Autodesk Fusion 360 part; units mm, degrees
(part 11 of 14)
  line L7370 (-262.9775, 77.7875) -> (-273.976, 77.7875)
  line L7371 (-273.976, 77.7875) -> (-279.4753, 68.2625)
  line L7372 (-279.4753, 68.2625) -> (-273.976, 58.7375)
  line L7373 (-273.976, 58.7375) -> (-262.9775, 58.7375)
  line L7374 (-257.4782, 68.2625) -> (-262.9775, 77.7875)
  line L7375 (-262.9775, 58.7375) -> (-257.4782, 68.2625)
  line L7376 (-243.7301, 88.9) -> (-254.7286, 88.9)
  line L7377 (-254.7286, 88.9) -> (-260.2278, 79.375)
  line L7378 (-260.2278, 79.375) -> (-254.7286, 69.85)
  line L7379 (-254.7286, 69.85) -> (-243.7301, 69.85)
  line L7380 (-238.2308, 79.375) -> (-243.7301, 88.9)
  line L7381 (-243.7301, 69.85) -> (-238.2308, 79.375)
  line L7382 (-224.4826, 100.0125) -> (-235.4812, 100.0125)
  line L7383 (-235.4812, 100.0125) -> (-240.9804, 90.4875)
  line L7384 (-240.9804, 90.4875) -> (-235.4812, 80.9625)
  line L7385 (-235.4812, 80.9625) -> (-224.4826, 80.9625)
  line L7386 (-218.9834, 90.4875) -> (-224.4826, 100.0125)
  line L7387 (-224.4826, 80.9625) -> (-218.9834, 90.4875)
  line L7388 (-205.2352, 111.125) -> (-216.2337, 111.125)
  line L7389 (-216.2337, 111.125) -> (-221.733, 101.6)
  line L7390 (-221.733, 101.6) -> (-216.2337, 92.075)
  line L7391 (-216.2337, 92.075) -> (-205.2352, 92.075)
  line L7392 (-199.736, 101.6) -> (-205.2352, 111.125)
  line L7393 (-205.2352, 92.075) -> (-199.736, 101.6)
  line L7394 (-185.9878, 122.2375) -> (-196.9863, 122.2375)
  line L7395 (-196.9863, 122.2375) -> (-202.4856, 112.7125)
  line L7396 (-202.4856, 112.7125) -> (-196.9863, 103.1875)
  line L7397 (-196.9863, 103.1875) -> (-185.9878, 103.1875)
  line L7398 (-180.4886, 112.7125) -> (-185.9878, 122.2375)
  line L7399 (-185.9878, 103.1875) -> (-180.4886, 112.7125)
  line L7400 (-166.7404, 133.35) -> (-177.7389, 133.35)
  line L7401 (-177.7389, 133.35) -> (-183.2382, 123.825)
  line L7402 (-183.2382, 123.825) -> (-177.7389, 114.3)
  line L7403 (-177.7389, 114.3) -> (-166.7404, 114.3)
  line L7404 (-161.2411, 123.825) -> (-166.7404, 133.35)
  line L7405 (-166.7404, 114.3) -> (-161.2411, 123.825)
  line L7406 (-147.493, 144.4625) -> (-158.4915, 144.4625)
  line L7407 (-158.4915, 144.4625) -> (-163.9908, 134.9375)
  line L7408 (-163.9908, 134.9375) -> (-158.4915, 125.4125)
  line L7409 (-158.4915, 125.4125) -> (-147.493, 125.4125)
  line L7410 (-141.9937, 134.9375) -> (-147.493, 144.4625)
  line L7411 (-147.493, 125.4125) -> (-141.9937, 134.9375)
  line L7412 (-128.2456, 155.575) -> (-139.2441, 155.575)
  line L7413 (-139.2441, 155.575) -> (-144.7434, 146.05)
  line L7414 (-144.7434, 146.05) -> (-139.2441, 136.525)
  line L7415 (-139.2441, 136.525) -> (-128.2456, 136.525)
  line L7416 (-122.7463, 146.05) -> (-128.2456, 155.575)
  line L7417 (-128.2456, 136.525) -> (-122.7463, 146.05)
  line L7418 (-108.9982, 166.6875) -> (-119.9967, 166.6875)
  line L7419 (-119.9967, 166.6875) -> (-125.4959, 157.1625)
  line L7420 (-125.4959, 157.1625) -> (-119.9967, 147.6375)
  line L7421 (-119.9967, 147.6375) -> (-108.9982, 147.6375)
  line L7422 (-103.4989, 157.1625) -> (-108.9982, 166.6875)
  line L7423 (-108.9982, 147.6375) -> (-103.4989, 157.1625)
  line L7424 (-89.7507, 177.8) -> (-100.7493, 177.8)
  line L7425 (-100.7493, 177.8) -> (-106.2485, 168.275)
  line L7426 (-106.2485, 168.275) -> (-100.7493, 158.75)
  line L7427 (-100.7493, 158.75) -> (-89.7507, 158.75)
  line L7428 (-84.2515, 168.275) -> (-89.7507, 177.8)
  line L7429 (-89.7507, 158.75) -> (-84.2515, 168.275)
  line L7430 (-70.5033, 188.9125) -> (-81.5018, 188.9125)
  line L7431 (-81.5018, 188.9125) -> (-87.0011, 179.3875)
  line L7432 (-87.0011, 179.3875) -> (-81.5018, 169.8625)
  line L7433 (-81.5018, 169.8625) -> (-70.5033, 169.8625)
  line L7434 (-65.0041, 179.3875) -> (-70.5033, 188.9125)
  line L7435 (-70.5033, 169.8625) -> (-65.0041, 179.3875)
  line L7436 (-51.2559, 200.025) -> (-62.2544, 200.025)
  line L7437 (-62.2544, 200.025) -> (-67.7537, 190.5)
  line L7438 (-67.7537, 190.5) -> (-62.2544, 180.975)
  line L7439 (-62.2544, 180.975) -> (-51.2559, 180.975)
  line L7440 (-45.7566, 190.5) -> (-51.2559, 200.025)
  line L7441 (-51.2559, 180.975) -> (-45.7566, 190.5)
  line L7442 (-32.0085, 211.1375) -> (-43.007, 211.1375)
  line L7443 (-43.007, 211.1375) -> (-48.5063, 201.6125)
  line L7444 (-48.5063, 201.6125) -> (-43.007, 192.0875)
  line L7445 (-43.007, 192.0875) -> (-32.0085, 192.0875)
  line L7446 (-26.5092, 201.6125) -> (-32.0085, 211.1375)
  line L7447 (-32.0085, 192.0875) -> (-26.5092, 201.6125)
  line L7448 (-12.7611, 222.25) -> (-23.7596, 222.25)
  line L7449 (-23.7596, 222.25) -> (-29.2589, 212.725)
  line L7450 (-29.2589, 212.725) -> (-23.7596, 203.2)
  line L7451 (-23.7596, 203.2) -> (-12.7611, 203.2)
  line L7452 (-7.2618, 212.725) -> (-12.7611, 222.25)
  line L7453 (-12.7611, 203.2) -> (-7.2618, 212.725)
  line L7454 (6.4863, 233.3625) -> (-4.5122, 233.3625)
  line L7455 (-4.5122, 233.3625) -> (-10.0114, 223.8375)
  line L7456 (-10.0114, 223.8375) -> (-4.5122, 214.3125)
  line L7457 (-4.5122, 214.3125) -> (6.4863, 214.3125)
  line L7458 (11.9856, 223.8375) -> (6.4863, 233.3625)
  line L7459 (6.4863, 214.3125) -> (11.9856, 223.8375)
  line L7460 (25.7337, 244.475) -> (14.7352, 244.475)
  line L7461 (14.7352, 244.475) -> (9.236, 234.95)
  line L7462 (9.236, 234.95) -> (14.7352, 225.425)
  line L7463 (14.7352, 225.425) -> (25.7337, 225.425)
  line L7464 (31.233, 234.95) -> (25.7337, 244.475)
  line L7465 (25.7337, 225.425) -> (31.233, 234.95)
  line L7466 (44.9812, 255.5875) -> (33.9826, 255.5875)
  line L7467 (33.9826, 255.5875) -> (28.4834, 246.0625)
  line L7468 (28.4834, 246.0625) -> (33.9826, 236.5375)
  line L7469 (33.9826, 236.5375) -> (44.9812, 236.5375)
  line L7470 (50.4804, 246.0625) -> (44.9812, 255.5875)
  line L7471 (44.9812, 236.5375) -> (50.4804, 246.0625)
  line L7472 (64.2286, 266.7) -> (53.2301, 266.7)
  line L7473 (53.2301, 266.7) -> (47.7308, 257.175)
  line L7474 (47.7308, 257.175) -> (53.2301, 247.65)
  line L7475 (53.2301, 247.65) -> (64.2286, 247.65)
  line L7476 (69.7278, 257.175) -> (64.2286, 266.7)
  line L7477 (64.2286, 247.65) -> (69.7278, 257.175)
  line L7478 (83.476, 277.8125) -> (72.4775, 277.8125)
  line L7479 (72.4775, 277.8125) -> (66.9782, 268.2875)
  line L7480 (66.9782, 268.2875) -> (72.4775, 258.7625)
  line L7481 (72.4775, 258.7625) -> (83.476, 258.7625)
  line L7482 (88.9753, 268.2875) -> (83.476, 277.8125)
  line L7483 (83.476, 258.7625) -> (88.9753, 268.2875)
  line L7484 (102.7234, 288.925) -> (91.7249, 288.925)
  line L7485 (91.7249, 288.925) -> (86.2256, 279.4)
  line L7486 (86.2256, 279.4) -> (91.7249, 269.875)
  line L7487 (91.7249, 269.875) -> (102.7234, 269.875)
  line L7488 (108.2227, 279.4) -> (102.7234, 288.925)
  line L7489 (102.7234, 269.875) -> (108.2227, 279.4)
  line L7490 (121.9708, 300.0375) -> (110.9723, 300.0375)
  line L7491 (110.9723, 300.0375) -> (105.473, 290.5125)
  line L7492 (105.473, 290.5125) -> (110.9723, 280.9875)
  line L7493 (110.9723, 280.9875) -> (121.9708, 280.9875)
  line L7494 (127.4701, 290.5125) -> (121.9708, 300.0375)
  line L7495 (121.9708, 280.9875) -> (127.4701, 290.5125)
  line L7496 (141.2182, 311.15) -> (130.2197, 311.15)
  line L7497 (130.2197, 311.15) -> (124.7205, 301.625)
  line L7498 (124.7205, 301.625) -> (130.2197, 292.1)
  line L7499 (130.2197, 292.1) -> (141.2182, 292.1)
  line L7500 (146.7175, 301.625) -> (141.2182, 311.15)
  line L7501 (141.2182, 292.1) -> (146.7175, 301.625)
  line L7502 (160.4657, 322.2625) -> (149.4671, 322.2625)
  line L7503 (149.4671, 322.2625) -> (143.9679, 312.7375)
  line L7504 (143.9679, 312.7375) -> (149.4671, 303.2125)
  line L7505 (149.4671, 303.2125) -> (160.4657, 303.2125)
  line L7506 (165.9649, 312.7375) -> (160.4657, 322.2625)
  line L7507 (160.4657, 303.2125) -> (165.9649, 312.7375)
  line L7508 (179.7131, 333.375) -> (168.7145, 333.375)
  line L7509 (168.7145, 333.375) -> (163.2153, 323.85)
  line L7510 (163.2153, 323.85) -> (168.7145, 314.325)
  line L7511 (168.7145, 314.325) -> (179.7131, 314.325)
  line L7512 (185.2123, 323.85) -> (179.7131, 333.375)
  line L7513 (179.7131, 314.325) -> (185.2123, 323.85)
  line L7514 (198.9605, 344.4875) -> (187.962, 344.4875)
  line L7515 (187.962, 344.4875) -> (182.4627, 334.9625)
  line L7516 (182.4627, 334.9625) -> (187.962, 325.4375)
  line L7517 (187.962, 325.4375) -> (198.9605, 325.4375)
  line L7518 (204.4597, 334.9625) -> (198.9605, 344.4875)
  line L7519 (198.9605, 325.4375) -> (204.4597, 334.9625)
  line L7520 (218.2079, 355.6) -> (207.2094, 355.6)
  line L7521 (207.2094, 355.6) -> (201.7101, 346.075)
  line L7522 (201.7101, 346.075) -> (207.2094, 336.55)
  line L7523 (207.2094, 336.55) -> (218.2079, 336.55)
  line L7524 (223.7072, 346.075) -> (218.2079, 355.6)
  line L7525 (218.2079, 336.55) -> (223.7072, 346.075)
  line L7526 (237.4553, 366.7125) -> (226.4568, 366.7125)
  line L7527 (226.4568, 366.7125) -> (220.9575, 357.1875)
  line L7528 (220.9575, 357.1875) -> (226.4568, 347.6625)
  line L7529 (226.4568, 347.6625) -> (237.4553, 347.6625)
  line L7530 (242.9546, 357.1875) -> (237.4553, 366.7125)
  line L7531 (237.4553, 347.6625) -> (242.9546, 357.1875)
  line L7532 (256.7027, 377.825) -> (245.7042, 377.825)
  line L7533 (245.7042, 377.825) -> (240.2049, 368.3)
  line L7534 (240.2049, 368.3) -> (245.7042, 358.775)
  line L7535 (245.7042, 358.775) -> (256.7027, 358.775)
  line L7536 (262.202, 368.3) -> (256.7027, 377.825)
  line L7537 (256.7027, 358.775) -> (262.202, 368.3)
  line L7538 (275.9501, 388.9375) -> (264.9516, 388.9375)
  line L7539 (264.9516, 388.9375) -> (259.4524, 379.4125)
  line L7540 (259.4524, 379.4125) -> (264.9516, 369.8875)
  line L7541 (264.9516, 369.8875) -> (275.9501, 369.8875)
  line L7542 (281.4494, 379.4125) -> (275.9501, 388.9375)
  line L7543 (275.9501, 369.8875) -> (281.4494, 379.4125)
  line L7544 (295.1976, 400.05) -> (284.199, 400.05)
  line L7545 (284.199, 400.05) -> (278.6998, 390.525)
  line L7546 (278.6998, 390.525) -> (284.199, 381)
  line L7547 (284.199, 381) -> (295.1976, 381)
  line L7548 (300.6968, 390.525) -> (295.1976, 400.05)
  line L7549 (295.1976, 381) -> (300.6968, 390.525)
  line L7550 (314.445, 411.1625) -> (303.4464, 411.1625)
  line L7551 (303.4464, 411.1625) -> (297.9472, 401.6375)
  line L7552 (297.9472, 401.6375) -> (303.4464, 392.1125)
  line L7553 (303.4464, 392.1125) -> (314.445, 392.1125)
  line L7554 (319.9442, 401.6375) -> (314.445, 411.1625)
  line L7555 (314.445, 392.1125) -> (319.9442, 401.6375)
  line L7556 (333.6924, 422.275) -> (322.6939, 422.275)
  line L7557 (322.6939, 422.275) -> (317.1946, 412.75)
  line L7558 (317.1946, 412.75) -> (322.6939, 403.225)
  line L7559 (322.6939, 403.225) -> (333.6924, 403.225)
  line L7560 (339.1916, 412.75) -> (333.6924, 422.275)
  line L7561 (333.6924, 403.225) -> (339.1916, 412.75)
  line L7562 (352.9398, 433.3875) -> (341.9413, 433.3875)
  line L7563 (341.9413, 433.3875) -> (336.442, 423.8625)
  line L7564 (336.442, 423.8625) -> (341.9413, 414.3375)
  line L7565 (341.9413, 414.3375) -> (352.9398, 414.3375)
  line L7566 (358.4391, 423.8625) -> (352.9398, 433.3875)
  line L7567 (352.9398, 414.3375) -> (358.4391, 423.8625)
  line L7568 (372.1872, 444.5) -> (361.1887, 444.5)
  line L7569 (361.1887, 444.5) -> (355.6894, 434.975)
  line L7570 (355.6894, 434.975) -> (361.1887, 425.45)
  line L7571 (361.1887, 425.45) -> (372.1872, 425.45)
  line L7572 (377.6865, 434.975) -> (372.1872, 444.5)
  line L7573 (372.1872, 425.45) -> (377.6865, 434.975)
  line L7574 (-782.6577, -200.025) -> (-793.6562, -200.025)
  line L7575 (-793.6562, -200.025) -> (-799.1554, -209.55)
  line L7576 (-799.1554, -209.55) -> (-793.6562, -219.075)
  line L7577 (-793.6562, -219.075) -> (-782.6577, -219.075)
  line L7578 (-777.1584, -209.55) -> (-782.6577, -200.025)
  line L7579 (-782.6577, -219.075) -> (-777.1584, -209.55)
  line L7580 (-763.4102, -188.9125) -> (-774.4088, -188.9125)
  line L7581 (-774.4088, -188.9125) -> (-779.908, -198.4375)
  line L7582 (-779.908, -198.4375) -> (-774.4088, -207.9625)
  line L7583 (-774.4088, -207.9625) -> (-763.4102, -207.9625)
  line L7584 (-757.911, -198.4375) -> (-763.4102, -188.9125)
  line L7585 (-763.4102, -207.9625) -> (-757.911, -198.4375)
  line L7586 (-744.1628, -177.8) -> (-755.1614, -177.8)
  line L7587 (-755.1614, -177.8) -> (-760.6606, -187.325)
  line L7588 (-760.6606, -187.325) -> (-755.1614, -196.85)
  line L7589 (-755.1614, -196.85) -> (-744.1628, -196.85)
  line L7590 (-738.6636, -187.325) -> (-744.1628, -177.8)
  line L7591 (-744.1628, -196.85) -> (-738.6636, -187.325)
  line L7592 (-724.9154, -166.6875) -> (-735.9139, -166.6875)
  line L7593 (-735.9139, -166.6875) -> (-741.4132, -176.2125)
  line L7594 (-741.4132, -176.2125) -> (-735.9139, -185.7375)
  line L7595 (-735.9139, -185.7375) -> (-724.9154, -185.7375)
  line L7596 (-719.4162, -176.2125) -> (-724.9154, -166.6875)
  line L7597 (-724.9154, -185.7375) -> (-719.4162, -176.2125)
  line L7598 (-705.668, -155.575) -> (-716.6665, -155.575)
  line L7599 (-716.6665, -155.575) -> (-722.1658, -165.1)
  line L7600 (-722.1658, -165.1) -> (-716.6665, -174.625)
  line L7601 (-716.6665, -174.625) -> (-705.668, -174.625)
  line L7602 (-700.1687, -165.1) -> (-705.668, -155.575)
  line L7603 (-705.668, -174.625) -> (-700.1687, -165.1)
  line L7604 (-686.4206, -144.4625) -> (-697.4191, -144.4625)
  line L7605 (-697.4191, -144.4625) -> (-702.9184, -153.9875)
  line L7606 (-702.9184, -153.9875) -> (-697.4191, -163.5125)
  line L7607 (-697.4191, -163.5125) -> (-686.4206, -163.5125)
  line L7608 (-680.9213, -153.9875) -> (-686.4206, -144.4625)
  line L7609 (-686.4206, -163.5125) -> (-680.9213, -153.9875)
  line L7610 (-667.1732, -133.35) -> (-678.1717, -133.35)
  line L7611 (-678.1717, -133.35) -> (-683.671, -142.875)
  line L7612 (-683.671, -142.875) -> (-678.1717, -152.4)
  line L7613 (-678.1717, -152.4) -> (-667.1732, -152.4)
  line L7614 (-661.6739, -142.875) -> (-667.1732, -133.35)
  line L7615 (-667.1732, -152.4) -> (-661.6739, -142.875)
  line L7616 (-647.9258, -122.2375) -> (-658.9243, -122.2375)
  line L7617 (-658.9243, -122.2375) -> (-664.4235, -131.7625)
  line L7618 (-664.4235, -131.7625) -> (-658.9243, -141.2875)
  line L7619 (-658.9243, -141.2875) -> (-647.9258, -141.2875)
  line L7620 (-642.4265, -131.7625) -> (-647.9258, -122.2375)
  line L7621 (-647.9258, -141.2875) -> (-642.4265, -131.7625)
  line L7622 (-628.6783, -111.125) -> (-639.6769, -111.125)
  line L7623 (-639.6769, -111.125) -> (-645.1761, -120.65)
  line L7624 (-645.1761, -120.65) -> (-639.6769, -130.175)
  line L7625 (-639.6769, -130.175) -> (-628.6783, -130.175)
  line L7626 (-623.1791, -120.65) -> (-628.6783, -111.125)
  line L7627 (-628.6783, -130.175) -> (-623.1791, -120.65)
  line L7628 (-609.4309, -100.0125) -> (-620.4295, -100.0125)
  line L7629 (-620.4295, -100.0125) -> (-625.9287, -109.5375)
  line L7630 (-625.9287, -109.5375) -> (-620.4295, -119.0625)
  line L7631 (-620.4295, -119.0625) -> (-609.4309, -119.0625)
  line L7632 (-603.9317, -109.5375) -> (-609.4309, -100.0125)
  line L7633 (-609.4309, -119.0625) -> (-603.9317, -109.5375)
  line L7634 (-590.1835, -88.9) -> (-601.182, -88.9)
  line L7635 (-601.182, -88.9) -> (-606.6813, -98.425)
  line L7636 (-606.6813, -98.425) -> (-601.182, -107.95)
  line L7637 (-601.182, -107.95) -> (-590.1835, -107.95)
  line L7638 (-584.6843, -98.425) -> (-590.1835, -88.9)
  line L7639 (-590.1835, -107.95) -> (-584.6843, -98.425)
  line L7640 (-570.9361, -77.7875) -> (-581.9346, -77.7875)
  line L7641 (-581.9346, -77.7875) -> (-587.4339, -87.3125)
  line L7642 (-587.4339, -87.3125) -> (-581.9346, -96.8375)
  line L7643 (-581.9346, -96.8375) -> (-570.9361, -96.8375)
  line L7644 (-565.4368, -87.3125) -> (-570.9361, -77.7875)
  line L7645 (-570.9361, -96.8375) -> (-565.4368, -87.3125)
  line L7646 (-551.6887, -66.675) -> (-562.6872, -66.675)
  line L7647 (-562.6872, -66.675) -> (-568.1865, -76.2)
  line L7648 (-568.1865, -76.2) -> (-562.6872, -85.725)
  line L7649 (-562.6872, -85.725) -> (-551.6887, -85.725)
  line L7650 (-546.1894, -76.2) -> (-551.6887, -66.675)
  line L7651 (-551.6887, -85.725) -> (-546.1894, -76.2)
  line L7652 (-532.4413, -55.5625) -> (-543.4398, -55.5625)
  line L7653 (-543.4398, -55.5625) -> (-548.9391, -65.0875)
  line L7654 (-548.9391, -65.0875) -> (-543.4398, -74.6125)
  line L7655 (-543.4398, -74.6125) -> (-532.4413, -74.6125)
  line L7656 (-526.942, -65.0875) -> (-532.4413, -55.5625)
  line L7657 (-532.4413, -74.6125) -> (-526.942, -65.0875)
  line L7658 (-513.1939, -44.45) -> (-524.1924, -44.45)
  line L7659 (-524.1924, -44.45) -> (-529.6916, -53.975)
  line L7660 (-529.6916, -53.975) -> (-524.1924, -63.5)
  line L7661 (-524.1924, -63.5) -> (-513.1939, -63.5)
  line L7662 (-507.6946, -53.975) -> (-513.1939, -44.45)
  line L7663 (-513.1939, -63.5) -> (-507.6946, -53.975)
  line L7664 (-493.9464, -33.3375) -> (-504.945, -33.3375)
  line L7665 (-504.945, -33.3375) -> (-510.4442, -42.8625)
  line L7666 (-510.4442, -42.8625) -> (-504.945, -52.3875)
  line L7667 (-504.945, -52.3875) -> (-493.9464, -52.3875)
  line L7668 (-488.4472, -42.8625) -> (-493.9464, -33.3375)
  line L7669 (-493.9464, -52.3875) -> (-488.4472, -42.8625)
  line L7670 (-474.699, -22.225) -> (-485.6976, -22.225)
  line L7671 (-485.6976, -22.225) -> (-491.1968, -31.75)
  line L7672 (-491.1968, -31.75) -> (-485.6976, -41.275)
  line L7673 (-485.6976, -41.275) -> (-474.699, -41.275)
  line L7674 (-469.1998, -31.75) -> (-474.699, -22.225)
  line L7675 (-474.699, -41.275) -> (-469.1998, -31.75)
  line L7676 (-455.4516, -11.1125) -> (-466.4501, -11.1125)
  line L7677 (-466.4501, -11.1125) -> (-471.9494, -20.6375)
  line L7678 (-471.9494, -20.6375) -> (-466.4501, -30.1625)
  line L7679 (-466.4501, -30.1625) -> (-455.4516, -30.1625)
  line L7680 (-449.9524, -20.6375) -> (-455.4516, -11.1125)
  line L7681 (-455.4516, -30.1625) -> (-449.9524, -20.6375)
  line L7682 (-436.2042, 0) -> (-447.2027, 0)
  line L7683 (-447.2027, 0) -> (-452.702, -9.525)
  line L7684 (-452.702, -9.525) -> (-447.2027, -19.05)
  line L7685 (-447.2027, -19.05) -> (-436.2042, -19.05)
  line L7686 (-430.7049, -9.525) -> (-436.2042, 0)
  line L7687 (-436.2042, -19.05) -> (-430.7049, -9.525)
  line L7688 (-416.9568, 11.1125) -> (-427.9553, 11.1125)
  line L7689 (-427.9553, 11.1125) -> (-433.4546, 1.5875)
  line L7690 (-433.4546, 1.5875) -> (-427.9553, -7.9375)
  line L7691 (-427.9553, -7.9375) -> (-416.9568, -7.9375)
  line L7692 (-411.4575, 1.5875) -> (-416.9568, 11.1125)
  line L7693 (-416.9568, -7.9375) -> (-411.4575, 1.5875)
  line L7694 (-397.7094, 22.225) -> (-408.7079, 22.225)
  line L7695 (-408.7079, 22.225) -> (-414.2072, 12.7)
  line L7696 (-414.2072, 12.7) -> (-408.7079, 3.175)
  line L7697 (-408.7079, 3.175) -> (-397.7094, 3.175)
  line L7698 (-392.2101, 12.7) -> (-397.7094, 22.225)
  line L7699 (-397.7094, 3.175) -> (-392.2101, 12.7)
  line L7700 (-378.462, 33.3375) -> (-389.4605, 33.3375)
  line L7701 (-389.4605, 33.3375) -> (-394.9597, 23.8125)
  line L7702 (-394.9597, 23.8125) -> (-389.4605, 14.2875)
  line L7703 (-389.4605, 14.2875) -> (-378.462, 14.2875)
  line L7704 (-372.9627, 23.8125) -> (-378.462, 33.3375)
  line L7705 (-378.462, 14.2875) -> (-372.9627, 23.8125)
  line L7706 (-359.2145, 44.45) -> (-370.2131, 44.45)
  line L7707 (-370.2131, 44.45) -> (-375.7123, 34.925)
  line L7708 (-375.7123, 34.925) -> (-370.2131, 25.4)
  line L7709 (-370.2131, 25.4) -> (-359.2145, 25.4)
  line L7710 (-353.7153, 34.925) -> (-359.2145, 44.45)
  line L7711 (-359.2145, 25.4) -> (-353.7153, 34.925)
  line L7712 (-339.9671, 55.5625) -> (-350.9657, 55.5625)
  line L7713 (-350.9657, 55.5625) -> (-356.4649, 46.0375)
  line L7714 (-356.4649, 46.0375) -> (-350.9657, 36.5125)
  line L7715 (-350.9657, 36.5125) -> (-339.9671, 36.5125)
  line L7716 (-334.4679, 46.0375) -> (-339.9671, 55.5625)
  line L7717 (-339.9671, 36.5125) -> (-334.4679, 46.0375)
  line L7718 (-320.7197, 66.675) -> (-331.7182, 66.675)
  line L7719 (-331.7182, 66.675) -> (-337.2175, 57.15)
  line L7720 (-337.2175, 57.15) -> (-331.7182, 47.625)
  line L7721 (-331.7182, 47.625) -> (-320.7197, 47.625)
  line L7722 (-315.2205, 57.15) -> (-320.7197, 66.675)
  line L7723 (-320.7197, 47.625) -> (-315.2205, 57.15)
  line L7724 (-301.4723, 77.7875) -> (-312.4708, 77.7875)
  line L7725 (-312.4708, 77.7875) -> (-317.9701, 68.2625)
  line L7726 (-317.9701, 68.2625) -> (-312.4708, 58.7375)
  line L7727 (-312.4708, 58.7375) -> (-301.4723, 58.7375)
  line L7728 (-295.973, 68.2625) -> (-301.4723, 77.7875)
  line L7729 (-301.4723, 58.7375) -> (-295.973, 68.2625)
  line L7730 (-282.2249, 88.9) -> (-293.2234, 88.9)
  line L7731 (-293.2234, 88.9) -> (-298.7227, 79.375)
  line L7732 (-298.7227, 79.375) -> (-293.2234, 69.85)
  line L7733 (-293.2234, 69.85) -> (-282.2249, 69.85)
  line L7734 (-276.7256, 79.375) -> (-282.2249, 88.9)
  line L7735 (-282.2249, 69.85) -> (-276.7256, 79.375)
  line L7736 (-262.9775, 100.0125) -> (-273.976, 100.0125)
  line L7737 (-273.976, 100.0125) -> (-279.4753, 90.4875)
  line L7738 (-279.4753, 90.4875) -> (-273.976, 80.9625)
  line L7739 (-273.976, 80.9625) -> (-262.9775, 80.9625)
  line L7740 (-257.4782, 90.4875) -> (-262.9775, 100.0125)
  line L7741 (-262.9775, 80.9625) -> (-257.4782, 90.4875)
  line L7742 (-243.7301, 111.125) -> (-254.7286, 111.125)
  line L7743 (-254.7286, 111.125) -> (-260.2278, 101.6)
  line L7744 (-260.2278, 101.6) -> (-254.7286, 92.075)
  line L7745 (-254.7286, 92.075) -> (-243.7301, 92.075)
  line L7746 (-238.2308, 101.6) -> (-243.7301, 111.125)
  line L7747 (-243.7301, 92.075) -> (-238.2308, 101.6)
  line L7748 (-224.4826, 122.2375) -> (-235.4812, 122.2375)
  line L7749 (-235.4812, 122.2375) -> (-240.9804, 112.7125)
  line L7750 (-240.9804, 112.7125) -> (-235.4812, 103.1875)
  line L7751 (-235.4812, 103.1875) -> (-224.4826, 103.1875)
  line L7752 (-218.9834, 112.7125) -> (-224.4826, 122.2375)
  line L7753 (-224.4826, 103.1875) -> (-218.9834, 112.7125)
  line L7754 (-205.2352, 133.35) -> (-216.2337, 133.35)
  line L7755 (-216.2337, 133.35) -> (-221.733, 123.825)
  line L7756 (-221.733, 123.825) -> (-216.2337, 114.3)
  line L7757 (-216.2337, 114.3) -> (-205.2352, 114.3)
  line L7758 (-199.736, 123.825) -> (-205.2352, 133.35)
  line L7759 (-205.2352, 114.3) -> (-199.736, 123.825)
  line L7760 (-185.9878, 144.4625) -> (-196.9863, 144.4625)
  line L7761 (-196.9863, 144.4625) -> (-202.4856, 134.9375)
  line L7762 (-202.4856, 134.9375) -> (-196.9863, 125.4125)
  line L7763 (-196.9863, 125.4125) -> (-185.9878, 125.4125)
  line L7764 (-180.4886, 134.9375) -> (-185.9878, 144.4625)
  line L7765 (-185.9878, 125.4125) -> (-180.4886, 134.9375)
  line L7766 (-166.7404, 155.575) -> (-177.7389, 155.575)
  line L7767 (-177.7389, 155.575) -> (-183.2382, 146.05)
  line L7768 (-183.2382, 146.05) -> (-177.7389, 136.525)
  line L7769 (-177.7389, 136.525) -> (-166.7404, 136.525)
  line L7770 (-161.2411, 146.05) -> (-166.7404, 155.575)
  line L7771 (-166.7404, 136.525) -> (-161.2411, 146.05)
  line L7772 (-147.493, 166.6875) -> (-158.4915, 166.6875)
  line L7773 (-158.4915, 166.6875) -> (-163.9908, 157.1625)
  line L7774 (-163.9908, 157.1625) -> (-158.4915, 147.6375)
  line L7775 (-158.4915, 147.6375) -> (-147.493, 147.6375)
  line L7776 (-141.9937, 157.1625) -> (-147.493, 166.6875)
  line L7777 (-147.493, 147.6375) -> (-141.9937, 157.1625)
  line L7778 (-128.2456, 177.8) -> (-139.2441, 177.8)
  line L7779 (-139.2441, 177.8) -> (-144.7434, 168.275)
  line L7780 (-144.7434, 168.275) -> (-139.2441, 158.75)
  line L7781 (-139.2441, 158.75) -> (-128.2456, 158.75)
  line L7782 (-122.7463, 168.275) -> (-128.2456, 177.8)
  line L7783 (-128.2456, 158.75) -> (-122.7463, 168.275)
  line L7784 (-108.9982, 188.9125) -> (-119.9967, 188.9125)
  line L7785 (-119.9967, 188.9125) -> (-125.4959, 179.3875)
  line L7786 (-125.4959, 179.3875) -> (-119.9967, 169.8625)
  line L7787 (-119.9967, 169.8625) -> (-108.9982, 169.8625)
  line L7788 (-103.4989, 179.3875) -> (-108.9982, 188.9125)
  line L7789 (-108.9982, 169.8625) -> (-103.4989, 179.3875)
  line L7790 (-89.7507, 200.025) -> (-100.7493, 200.025)
  line L7791 (-100.7493, 200.025) -> (-106.2485, 190.5)
  line L7792 (-106.2485, 190.5) -> (-100.7493, 180.975)
  line L7793 (-100.7493, 180.975) -> (-89.7507, 180.975)
  line L7794 (-84.2515, 190.5) -> (-89.7507, 200.025)
  line L7795 (-89.7507, 180.975) -> (-84.2515, 190.5)
  line L7796 (-70.5033, 211.1375) -> (-81.5018, 211.1375)
  line L7797 (-81.5018, 211.1375) -> (-87.0011, 201.6125)
  line L7798 (-87.0011, 201.6125) -> (-81.5018, 192.0875)
  line L7799 (-81.5018, 192.0875) -> (-70.5033, 192.0875)
  line L7800 (-65.0041, 201.6125) -> (-70.5033, 211.1375)
  line L7801 (-70.5033, 192.0875) -> (-65.0041, 201.6125)
  line L7802 (-51.2559, 222.25) -> (-62.2544, 222.25)
  line L7803 (-62.2544, 222.25) -> (-67.7537, 212.725)
  line L7804 (-67.7537, 212.725) -> (-62.2544, 203.2)
  line L7805 (-62.2544, 203.2) -> (-51.2559, 203.2)
  line L7806 (-45.7566, 212.725) -> (-51.2559, 222.25)
  line L7807 (-51.2559, 203.2) -> (-45.7566, 212.725)
  line L7808 (-32.0085, 233.3625) -> (-43.007, 233.3625)
  line L7809 (-43.007, 233.3625) -> (-48.5063, 223.8375)
  line L7810 (-48.5063, 223.8375) -> (-43.007, 214.3125)
  line L7811 (-43.007, 214.3125) -> (-32.0085, 214.3125)
  line L7812 (-26.5092, 223.8375) -> (-32.0085, 233.3625)
  line L7813 (-32.0085, 214.3125) -> (-26.5092, 223.8375)
  line L7814 (-12.7611, 244.475) -> (-23.7596, 244.475)
  line L7815 (-23.7596, 244.475) -> (-29.2589, 234.95)
  line L7816 (-29.2589, 234.95) -> (-23.7596, 225.425)
  line L7817 (-23.7596, 225.425) -> (-12.7611, 225.425)
  line L7818 (-7.2618, 234.95) -> (-12.7611, 244.475)
  line L7819 (-12.7611, 225.425) -> (-7.2618, 234.95)
  line L7820 (6.4863, 255.5875) -> (-4.5122, 255.5875)
  line L7821 (-4.5122, 255.5875) -> (-10.0114, 246.0625)
  line L7822 (-10.0114, 246.0625) -> (-4.5122, 236.5375)
  line L7823 (-4.5122, 236.5375) -> (6.4863, 236.5375)
  line L7824 (11.9856, 246.0625) -> (6.4863, 255.5875)
  line L7825 (6.4863, 236.5375) -> (11.9856, 246.0625)
  line L7826 (25.7337, 266.7) -> (14.7352, 266.7)
  line L7827 (14.7352, 266.7) -> (9.236, 257.175)
  line L7828 (9.236, 257.175) -> (14.7352, 247.65)
  line L7829 (14.7352, 247.65) -> (25.7337, 247.65)
  line L7830 (31.233, 257.175) -> (25.7337, 266.7)
  line L7831 (25.7337, 247.65) -> (31.233, 257.175)
  line L7832 (44.9812, 277.8125) -> (33.9826, 277.8125)
  line L7833 (33.9826, 277.8125) -> (28.4834, 268.2875)
  line L7834 (28.4834, 268.2875) -> (33.9826, 258.7625)
  line L7835 (33.9826, 258.7625) -> (44.9812, 258.7625)
  line L7836 (50.4804, 268.2875) -> (44.9812, 277.8125)
  line L7837 (44.9812, 258.7625) -> (50.4804, 268.2875)
  line L7838 (64.2286, 288.925) -> (53.2301, 288.925)
  line L7839 (53.2301, 288.925) -> (47.7308, 279.4)
  line L7840 (47.7308, 279.4) -> (53.2301, 269.875)
  line L7841 (53.2301, 269.875) -> (64.2286, 269.875)
  line L7842 (69.7278, 279.4) -> (64.2286, 288.925)
  line L7843 (64.2286, 269.875) -> (69.7278, 279.4)
  line L7844 (83.476, 300.0375) -> (72.4775, 300.0375)
  line L7845 (72.4775, 300.0375) -> (66.9782, 290.5125)
  line L7846 (66.9782, 290.5125) -> (72.4775, 280.9875)
  line L7847 (72.4775, 280.9875) -> (83.476, 280.9875)
  line L7848 (88.9753, 290.5125) -> (83.476, 300.0375)
  line L7849 (83.476, 280.9875) -> (88.9753, 290.5125)
  line L7850 (102.7234, 311.15) -> (91.7249, 311.15)
  line L7851 (91.7249, 311.15) -> (86.2256, 301.625)
  line L7852 (86.2256, 301.625) -> (91.7249, 292.1)
  line L7853 (91.7249, 292.1) -> (102.7234, 292.1)
  line L7854 (108.2227, 301.625) -> (102.7234, 311.15)
  line L7855 (102.7234, 292.1) -> (108.2227, 301.625)
  line L7856 (121.9708, 322.2625) -> (110.9723, 322.2625)
  line L7857 (110.9723, 322.2625) -> (105.473, 312.7375)
  line L7858 (105.473, 312.7375) -> (110.9723, 303.2125)
  line L7859 (110.9723, 303.2125) -> (121.9708, 303.2125)
  line L7860 (127.4701, 312.7375) -> (121.9708, 322.2625)
  line L7861 (121.9708, 303.2125) -> (127.4701, 312.7375)
  line L7862 (141.2182, 333.375) -> (130.2197, 333.375)
  line L7863 (130.2197, 333.375) -> (124.7205, 323.85)
  line L7864 (124.7205, 323.85) -> (130.2197, 314.325)
  line L7865 (130.2197, 314.325) -> (141.2182, 314.325)
  line L7866 (146.7175, 323.85) -> (141.2182, 333.375)
  line L7867 (141.2182, 314.325) -> (146.7175, 323.85)
  line L7868 (160.4657, 344.4875) -> (149.4671, 344.4875)
  line L7869 (149.4671, 344.4875) -> (143.9679, 334.9625)
  line L7870 (143.9679, 334.9625) -> (149.4671, 325.4375)
  line L7871 (149.4671, 325.4375) -> (160.4657, 325.4375)
  line L7872 (165.9649, 334.9625) -> (160.4657, 344.4875)
  line L7873 (160.4657, 325.4375) -> (165.9649, 334.9625)
  line L7874 (179.7131, 355.6) -> (168.7145, 355.6)
  line L7875 (168.7145, 355.6) -> (163.2153, 346.075)
  line L7876 (163.2153, 346.075) -> (168.7145, 336.55)
  line L7877 (168.7145, 336.55) -> (179.7131, 336.55)
  line L7878 (185.2123, 346.075) -> (179.7131, 355.6)
  line L7879 (179.7131, 336.55) -> (185.2123, 346.075)
  line L7880 (198.9605, 366.7125) -> (187.962, 366.7125)
  line L7881 (187.962, 366.7125) -> (182.4627, 357.1875)
  line L7882 (182.4627, 357.1875) -> (187.962, 347.6625)
  line L7883 (187.962, 347.6625) -> (198.9605, 347.6625)
  line L7884 (204.4597, 357.1875) -> (198.9605, 366.7125)
  line L7885 (198.9605, 347.6625) -> (204.4597, 357.1875)
  line L7886 (218.2079, 377.825) -> (207.2094, 377.825)
  line L7887 (207.2094, 377.825) -> (201.7101, 368.3)
  line L7888 (201.7101, 368.3) -> (207.2094, 358.775)
  line L7889 (207.2094, 358.775) -> (218.2079, 358.775)
  line L7890 (223.7072, 368.3) -> (218.2079, 377.825)
  line L7891 (218.2079, 358.775) -> (223.7072, 368.3)
  line L7892 (237.4553, 388.9375) -> (226.4568, 388.9375)
  line L7893 (226.4568, 388.9375) -> (220.9575, 379.4125)
  line L7894 (220.9575, 379.4125) -> (226.4568, 369.8875)
  line L7895 (226.4568, 369.8875) -> (237.4553, 369.8875)
  line L7896 (242.9546, 379.4125) -> (237.4553, 388.9375)
  line L7897 (237.4553, 369.8875) -> (242.9546, 379.4125)
  line L7898 (256.7027, 400.05) -> (245.7042, 400.05)
  line L7899 (245.7042, 400.05) -> (240.2049, 390.525)
  line L7900 (240.2049, 390.525) -> (245.7042, 381)
  line L7901 (245.7042, 381) -> (256.7027, 381)
  line L7902 (262.202, 390.525) -> (256.7027, 400.05)
  line L7903 (256.7027, 381) -> (262.202, 390.525)
  line L7904 (275.9501, 411.1625) -> (264.9516, 411.1625)
  line L7905 (264.9516, 411.1625) -> (259.4524, 401.6375)
  line L7906 (259.4524, 401.6375) -> (264.9516, 392.1125)
  line L7907 (264.9516, 392.1125) -> (275.9501, 392.1125)
  line L7908 (281.4494, 401.6375) -> (275.9501, 411.1625)
  line L7909 (275.9501, 392.1125) -> (281.4494, 401.6375)
  line L7910 (295.1976, 422.275) -> (284.199, 422.275)
  line L7911 (284.199, 422.275) -> (278.6998, 412.75)
  line L7912 (278.6998, 412.75) -> (284.199, 403.225)
  line L7913 (284.199, 403.225) -> (295.1976, 403.225)
  line L7914 (300.6968, 412.75) -> (295.1976, 422.275)
  line L7915 (295.1976, 403.225) -> (300.6968, 412.75)
  line L7916 (314.445, 433.3875) -> (303.4464, 433.3875)
  line L7917 (303.4464, 433.3875) -> (297.9472, 423.8625)
  line L7918 (297.9472, 423.8625) -> (303.4464, 414.3375)
  line L7919 (303.4464, 414.3375) -> (314.445, 414.3375)
  line L7920 (319.9442, 423.8625) -> (314.445, 433.3875)
  line L7921 (314.445, 414.3375) -> (319.9442, 423.8625)
  line L7922 (333.6924, 444.5) -> (322.6939, 444.5)
  line L7923 (322.6939, 444.5) -> (317.1946, 434.975)
  line L7924 (317.1946, 434.975) -> (322.6939, 425.45)
  line L7925 (322.6939, 425.45) -> (333.6924, 425.45)
  line L7926 (339.1916, 434.975) -> (333.6924, 444.5)
  line L7927 (333.6924, 425.45) -> (339.1916, 434.975)
  line L7928 (352.9398, 455.6125) -> (341.9413, 455.6125)
  line L7929 (341.9413, 455.6125) -> (336.442, 446.0875)
  line L7930 (336.442, 446.0875) -> (341.9413, 436.5625)
  line L7931 (341.9413, 436.5625) -> (352.9398, 436.5625)
  line L7932 (358.4391, 446.0875) -> (352.9398, 455.6125)
  line L7933 (352.9398, 436.5625) -> (358.4391, 446.0875)
  line L7934 (-801.9051, -188.9125) -> (-812.9036, -188.9125)
  line L7935 (-812.9036, -188.9125) -> (-818.4029, -198.4375)
  line L7936 (-818.4029, -198.4375) -> (-812.9036, -207.9625)
  line L7937 (-812.9036, -207.9625) -> (-801.9051, -207.9625)
  line L7938 (-796.4058, -198.4375) -> (-801.9051, -188.9125)
  line L7939 (-801.9051, -207.9625) -> (-796.4058, -198.4375)
  line L7940 (-782.6577, -177.8) -> (-793.6562, -177.8)
  line L7941 (-793.6562, -177.8) -> (-799.1554, -187.325)
  line L7942 (-799.1554, -187.325) -> (-793.6562, -196.85)
  line L7943 (-793.6562, -196.85) -> (-782.6577, -196.85)
  line L7944 (-777.1584, -187.325) -> (-782.6577, -177.8)
  line L7945 (-782.6577, -196.85) -> (-777.1584, -187.325)
  line L7946 (-763.4102, -166.6875) -> (-774.4088, -166.6875)
  line L7947 (-774.4088, -166.6875) -> (-779.908, -176.2125)
  line L7948 (-779.908, -176.2125) -> (-774.4088, -185.7375)
  line L7949 (-774.4088, -185.7375) -> (-763.4102, -185.7375)
  line L7950 (-757.911, -176.2125) -> (-763.4102, -166.6875)
  line L7951 (-763.4102, -185.7375) -> (-757.911, -176.2125)
  line L7952 (-744.1628, -155.575) -> (-755.1614, -155.575)
  line L7953 (-755.1614, -155.575) -> (-760.6606, -165.1)
  line L7954 (-760.6606, -165.1) -> (-755.1614, -174.625)
  line L7955 (-755.1614, -174.625) -> (-744.1628, -174.625)
  line L7956 (-738.6636, -165.1) -> (-744.1628, -155.575)
  line L7957 (-744.1628, -174.625) -> (-738.6636, -165.1)
  line L7958 (-724.9154, -144.4625) -> (-735.9139, -144.4625)
  line L7959 (-735.9139, -144.4625) -> (-741.4132, -153.9875)
  line L7960 (-741.4132, -153.9875) -> (-735.9139, -163.5125)
  line L7961 (-735.9139, -163.5125) -> (-724.9154, -163.5125)
  line L7962 (-719.4162, -153.9875) -> (-724.9154, -144.4625)
  line L7963 (-724.9154, -163.5125) -> (-719.4162, -153.9875)
  line L7964 (-705.668, -133.35) -> (-716.6665, -133.35)
  line L7965 (-716.6665, -133.35) -> (-722.1658, -142.875)
  line L7966 (-722.1658, -142.875) -> (-716.6665, -152.4)
  line L7967 (-716.6665, -152.4) -> (-705.668, -152.4)
  line L7968 (-700.1687, -142.875) -> (-705.668, -133.35)
  line L7969 (-705.668, -152.4) -> (-700.1687, -142.875)
  line L7970 (-686.4206, -122.2375) -> (-697.4191, -122.2375)
  line L7971 (-697.4191, -122.2375) -> (-702.9184, -131.7625)
  line L7972 (-702.9184, -131.7625) -> (-697.4191, -141.2875)
  line L7973 (-697.4191, -141.2875) -> (-686.4206, -141.2875)
  line L7974 (-680.9213, -131.7625) -> (-686.4206, -122.2375)
  line L7975 (-686.4206, -141.2875) -> (-680.9213, -131.7625)
  line L7976 (-667.1732, -111.125) -> (-678.1717, -111.125)
  line L7977 (-678.1717, -111.125) -> (-683.671, -120.65)
  line L7978 (-683.671, -120.65) -> (-678.1717, -130.175)
  line L7979 (-678.1717, -130.175) -> (-667.1732, -130.175)
  line L7980 (-661.6739, -120.65) -> (-667.1732, -111.125)
  line L7981 (-667.1732, -130.175) -> (-661.6739, -120.65)
  line L7982 (-647.9258, -100.0125) -> (-658.9243, -100.0125)
  line L7983 (-658.9243, -100.0125) -> (-664.4235, -109.5375)
  line L7984 (-664.4235, -109.5375) -> (-658.9243, -119.0625)
  line L7985 (-658.9243, -119.0625) -> (-647.9258, -119.0625)
  line L7986 (-642.4265, -109.5375) -> (-647.9258, -100.0125)
  line L7987 (-647.9258, -119.0625) -> (-642.4265, -109.5375)
  line L7988 (-628.6783, -88.9) -> (-639.6769, -88.9)
  line L7989 (-639.6769, -88.9) -> (-645.1761, -98.425)
  line L7990 (-645.1761, -98.425) -> (-639.6769, -107.95)
  line L7991 (-639.6769, -107.95) -> (-628.6783, -107.95)
  line L7992 (-623.1791, -98.425) -> (-628.6783, -88.9)
  line L7993 (-628.6783, -107.95) -> (-623.1791, -98.425)
  line L7994 (-609.4309, -77.7875) -> (-620.4295, -77.7875)
  line L7995 (-620.4295, -77.7875) -> (-625.9287, -87.3125)
  line L7996 (-625.9287, -87.3125) -> (-620.4295, -96.8375)
  line L7997 (-620.4295, -96.8375) -> (-609.4309, -96.8375)
  line L7998 (-603.9317, -87.3125) -> (-609.4309, -77.7875)
  line L7999 (-609.4309, -96.8375) -> (-603.9317, -87.3125)
  line L8000 (-590.1835, -66.675) -> (-601.182, -66.675)
  line L8001 (-601.182, -66.675) -> (-606.6813, -76.2)
  line L8002 (-606.6813, -76.2) -> (-601.182, -85.725)
  line L8003 (-601.182, -85.725) -> (-590.1835, -85.725)
  line L8004 (-584.6843, -76.2) -> (-590.1835, -66.675)
  line L8005 (-590.1835, -85.725) -> (-584.6843, -76.2)
  line L8006 (-570.9361, -55.5625) -> (-581.9346, -55.5625)
  line L8007 (-581.9346, -55.5625) -> (-587.4339, -65.0875)
  line L8008 (-587.4339, -65.0875) -> (-581.9346, -74.6125)
  line L8009 (-581.9346, -74.6125) -> (-570.9361, -74.6125)
  line L8010 (-565.4368, -65.0875) -> (-570.9361, -55.5625)
  line L8011 (-570.9361, -74.6125) -> (-565.4368, -65.0875)
  line L8012 (-551.6887, -44.45) -> (-562.6872, -44.45)
  line L8013 (-562.6872, -44.45) -> (-568.1865, -53.975)
  line L8014 (-568.1865, -53.975) -> (-562.6872, -63.5)
  line L8015 (-562.6872, -63.5) -> (-551.6887, -63.5)
  line L8016 (-546.1894, -53.975) -> (-551.6887, -44.45)
  line L8017 (-551.6887, -63.5) -> (-546.1894, -53.975)
  line L8018 (-532.4413, -33.3375) -> (-543.4398, -33.3375)
  line L8019 (-543.4398, -33.3375) -> (-548.9391, -42.8625)
  line L8020 (-548.9391, -42.8625) -> (-543.4398, -52.3875)
  line L8021 (-543.4398, -52.3875) -> (-532.4413, -52.3875)
  line L8022 (-526.942, -42.8625) -> (-532.4413, -33.3375)
  line L8023 (-532.4413, -52.3875) -> (-526.942, -42.8625)
  line L8024 (-513.1939, -22.225) -> (-524.1924, -22.225)
  line L8025 (-524.1924, -22.225) -> (-529.6916, -31.75)
  line L8026 (-529.6916, -31.75) -> (-524.1924, -41.275)
  line L8027 (-524.1924, -41.275) -> (-513.1939, -41.275)
  line L8028 (-507.6946, -31.75) -> (-513.1939, -22.225)
  line L8029 (-513.1939, -41.275) -> (-507.6946, -31.75)
  line L8030 (-493.9464, -11.1125) -> (-504.945, -11.1125)
  line L8031 (-504.945, -11.1125) -> (-510.4442, -20.6375)
  line L8032 (-510.4442, -20.6375) -> (-504.945, -30.1625)
  line L8033 (-504.945, -30.1625) -> (-493.9464, -30.1625)
  line L8034 (-488.4472, -20.6375) -> (-493.9464, -11.1125)
  line L8035 (-493.9464, -30.1625) -> (-488.4472, -20.6375)
  line L8036 (-474.699, 0) -> (-485.6976, 0)
  line L8037 (-485.6976, 0) -> (-491.1968, -9.525)
  line L8038 (-491.1968, -9.525) -> (-485.6976, -19.05)
  line L8039 (-485.6976, -19.05) -> (-474.699, -19.05)
  line L8040 (-469.1998, -9.525) -> (-474.699, 0)
  line L8041 (-474.699, -19.05) -> (-469.1998, -9.525)
  line L8042 (-455.4516, 11.1125) -> (-466.4501, 11.1125)
  line L8043 (-466.4501, 11.1125) -> (-471.9494, 1.5875)
  line L8044 (-471.9494, 1.5875) -> (-466.4501, -7.9375)
  line L8045 (-466.4501, -7.9375) -> (-455.4516, -7.9375)
  line L8046 (-449.9524, 1.5875) -> (-455.4516, 11.1125)
  line L8047 (-455.4516, -7.9375) -> (-449.9524, 1.5875)
  line L8048 (-436.2042, 22.225) -> (-447.2027, 22.225)
  line L8049 (-447.2027, 22.225) -> (-452.702, 12.7)
  line L8050 (-452.702, 12.7) -> (-447.2027, 3.175)
  line L8051 (-447.2027, 3.175) -> (-436.2042, 3.175)
  line L8052 (-430.7049, 12.7) -> (-436.2042, 22.225)
  line L8053 (-436.2042, 3.175) -> (-430.7049, 12.7)
  line L8054 (-416.9568, 33.3375) -> (-427.9553, 33.3375)
  line L8055 (-427.9553, 33.3375) -> (-433.4546, 23.8125)
  line L8056 (-433.4546, 23.8125) -> (-427.9553, 14.2875)
  line L8057 (-427.9553, 14.2875) -> (-416.9568, 14.2875)
  line L8058 (-411.4575, 23.8125) -> (-416.9568, 33.3375)
  line L8059 (-416.9568, 14.2875) -> (-411.4575, 23.8125)
  line L8060 (-397.7094, 44.45) -> (-408.7079, 44.45)
  line L8061 (-408.7079, 44.45) -> (-414.2072, 34.925)
  line L8062 (-414.2072, 34.925) -> (-408.7079, 25.4)
  line L8063 (-408.7079, 25.4) -> (-397.7094, 25.4)
  line L8064 (-392.2101, 34.925) -> (-397.7094, 44.45)
  line L8065 (-397.7094, 25.4) -> (-392.2101, 34.925)
  line L8066 (-378.462, 55.5625) -> (-389.4605, 55.5625)
  line L8067 (-389.4605, 55.5625) -> (-394.9597, 46.0375)
  line L8068 (-394.9597, 46.0375) -> (-389.4605, 36.5125)
  line L8069 (-389.4605, 36.5125) -> (-378.462, 36.5125)
  line L8070 (-372.9627, 46.0375) -> (-378.462, 55.5625)
  line L8071 (-378.462, 36.5125) -> (-372.9627, 46.0375)
  line L8072 (-359.2145, 66.675) -> (-370.2131, 66.675)
  line L8073 (-370.2131, 66.675) -> (-375.7123, 57.15)
  line L8074 (-375.7123, 57.15) -> (-370.2131, 47.625)
  line L8075 (-370.2131, 47.625) -> (-359.2145, 47.625)
  line L8076 (-353.7153, 57.15) -> (-359.2145, 66.675)
  line L8077 (-359.2145, 47.625) -> (-353.7153, 57.15)
  line L8078 (-339.9671, 77.7875) -> (-350.9657, 77.7875)
  line L8079 (-350.9657, 77.7875) -> (-356.4649, 68.2625)
  line L8080 (-356.4649, 68.2625) -> (-350.9657, 58.7375)
  line L8081 (-350.9657, 58.7375) -> (-339.9671, 58.7375)
  line L8082 (-334.4679, 68.2625) -> (-339.9671, 77.7875)
  line L8083 (-339.9671, 58.7375) -> (-334.4679, 68.2625)
  line L8084 (-320.7197, 88.9) -> (-331.7182, 88.9)
  line L8085 (-331.7182, 88.9) -> (-337.2175, 79.375)
  line L8086 (-337.2175, 79.375) -> (-331.7182, 69.85)
  line L8087 (-331.7182, 69.85) -> (-320.7197, 69.85)
  line L8088 (-315.2205, 79.375) -> (-320.7197, 88.9)
  line L8089 (-320.7197, 69.85) -> (-315.2205, 79.375)
  line L8090 (-301.4723, 100.0125) -> (-312.4708, 100.0125)
  line L8091 (-312.4708, 100.0125) -> (-317.9701, 90.4875)
  line L8092 (-317.9701, 90.4875) -> (-312.4708, 80.9625)
  line L8093 (-312.4708, 80.9625) -> (-301.4723, 80.9625)
  line L8094 (-295.973, 90.4875) -> (-301.4723, 100.0125)
  line L8095 (-301.4723, 80.9625) -> (-295.973, 90.4875)
  line L8096 (-282.2249, 111.125) -> (-293.2234, 111.125)
  line L8097 (-293.2234, 111.125) -> (-298.7227, 101.6)
  line L8098 (-298.7227, 101.6) -> (-293.2234, 92.075)
  line L8099 (-293.2234, 92.075) -> (-282.2249, 92.075)
  line L8100 (-276.7256, 101.6) -> (-282.2249, 111.125)
  line L8101 (-282.2249, 92.075) -> (-276.7256, 101.6)
  line L8102 (-262.9775, 122.2375) -> (-273.976, 122.2375)
  line L8103 (-273.976, 122.2375) -> (-279.4753, 112.7125)
  line L8104 (-279.4753, 112.7125) -> (-273.976, 103.1875)
  line L8105 (-273.976, 103.1875) -> (-262.9775, 103.1875)
  line L8106 (-257.4782, 112.7125) -> (-262.9775, 122.2375)
  line L8107 (-262.9775, 103.1875) -> (-257.4782, 112.7125)
  line L8108 (-243.7301, 133.35) -> (-254.7286, 133.35)
  line L8109 (-254.7286, 133.35) -> (-260.2278, 123.825)
  line L8110 (-260.2278, 123.825) -> (-254.7286, 114.3)
  line L8111 (-254.7286, 114.3) -> (-243.7301, 114.3)
  line L8112 (-238.2308, 123.825) -> (-243.7301, 133.35)
  line L8113 (-243.7301, 114.3) -> (-238.2308, 123.825)
  line L8114 (-224.4826, 144.4625) -> (-235.4812, 144.4625)
  line L8115 (-235.4812, 144.4625) -> (-240.9804, 134.9375)
  line L8116 (-240.9804, 134.9375) -> (-235.4812, 125.4125)
  line L8117 (-235.4812, 125.4125) -> (-224.4826, 125.4125)
  line L8118 (-218.9834, 134.9375) -> (-224.4826, 144.4625)
  line L8119 (-224.4826, 125.4125) -> (-218.9834, 134.9375)
  line L8120 (-205.2352, 155.575) -> (-216.2337, 155.575)
  line L8121 (-216.2337, 155.575) -> (-221.733, 146.05)
  line L8122 (-221.733, 146.05) -> (-216.2337, 136.525)
  line L8123 (-216.2337, 136.525) -> (-205.2352, 136.525)
  line L8124 (-199.736, 146.05) -> (-205.2352, 155.575)
  line L8125 (-205.2352, 136.525) -> (-199.736, 146.05)
  line L8126 (-185.9878, 166.6875) -> (-196.9863, 166.6875)
  line L8127 (-196.9863, 166.6875) -> (-202.4856, 157.1625)
  line L8128 (-202.4856, 157.1625) -> (-196.9863, 147.6375)
  line L8129 (-196.9863, 147.6375) -> (-185.9878, 147.6375)
  line L8130 (-180.4886, 157.1625) -> (-185.9878, 166.6875)
  line L8131 (-185.9878, 147.6375) -> (-180.4886, 157.1625)
  line L8132 (-166.7404, 177.8) -> (-177.7389, 177.8)
  line L8133 (-177.7389, 177.8) -> (-183.2382, 168.275)
  line L8134 (-183.2382, 168.275) -> (-177.7389, 158.75)
  line L8135 (-177.7389, 158.75) -> (-166.7404, 158.75)
  line L8136 (-161.2411, 168.275) -> (-166.7404, 177.8)
  line L8137 (-166.7404, 158.75) -> (-161.2411, 168.275)
  line L8138 (-147.493, 188.9125) -> (-158.4915, 188.9125)
  line L8139 (-158.4915, 188.9125) -> (-163.9908, 179.3875)
  line L8140 (-163.9908, 179.3875) -> (-158.4915, 169.8625)
  line L8141 (-158.4915, 169.8625) -> (-147.493, 169.8625)
  line L8142 (-141.9937, 179.3875) -> (-147.493, 188.9125)
  line L8143 (-147.493, 169.8625) -> (-141.9937, 179.3875)
  line L8144 (-128.2456, 200.025) -> (-139.2441, 200.025)
  line L8145 (-139.2441, 200.025) -> (-144.7434, 190.5)
  line L8146 (-144.7434, 190.5) -> (-139.2441, 180.975)
  line L8147 (-139.2441, 180.975) -> (-128.2456, 180.975)
  line L8148 (-122.7463, 190.5) -> (-128.2456, 200.025)
  line L8149 (-128.2456, 180.975) -> (-122.7463, 190.5)
  line L8150 (-108.9982, 211.1375) -> (-119.9967, 211.1375)
  line L8151 (-119.9967, 211.1375) -> (-125.4959, 201.6125)
  line L8152 (-125.4959, 201.6125) -> (-119.9967, 192.0875)
  line L8153 (-119.9967, 192.0875) -> (-108.9982, 192.0875)
  line L8154 (-103.4989, 201.6125) -> (-108.9982, 211.1375)
  line L8155 (-108.9982, 192.0875) -> (-103.4989, 201.6125)
  line L8156 (-89.7507, 222.25) -> (-100.7493, 222.25)
  line L8157 (-100.7493, 222.25) -> (-106.2485, 212.725)
  line L8158 (-106.2485, 212.725) -> (-100.7493, 203.2)
  line L8159 (-100.7493, 203.2) -> (-89.7507, 203.2)
  line L8160 (-84.2515, 212.725) -> (-89.7507, 222.25)
  line L8161 (-89.7507, 203.2) -> (-84.2515, 212.725)
  line L8162 (-70.5033, 233.3625) -> (-81.5018, 233.3625)
  line L8163 (-81.5018, 233.3625) -> (-87.0011, 223.8375)
  line L8164 (-87.0011, 223.8375) -> (-81.5018, 214.3125)
  line L8165 (-81.5018, 214.3125) -> (-70.5033, 214.3125)
  line L8166 (-65.0041, 223.8375) -> (-70.5033, 233.3625)
  line L8167 (-70.5033, 214.3125) -> (-65.0041, 223.8375)
  line L8168 (-51.2559, 244.475) -> (-62.2544, 244.475)
  line L8169 (-62.2544, 244.475) -> (-67.7537, 234.95)
  line L8170 (-67.7537, 234.95) -> (-62.2544, 225.425)
  line L8171 (-62.2544, 225.425) -> (-51.2559, 225.425)
  line L8172 (-45.7566, 234.95) -> (-51.2559, 244.475)
  line L8173 (-51.2559, 225.425) -> (-45.7566, 234.95)
  line L8174 (-32.0085, 255.5875) -> (-43.007, 255.5875)
  line L8175 (-43.007, 255.5875) -> (-48.5063, 246.0625)
  line L8176 (-48.5063, 246.0625) -> (-43.007, 236.5375)
  line L8177 (-43.007, 236.5375) -> (-32.0085, 236.5375)
  line L8178 (-26.5092, 246.0625) -> (-32.0085, 255.5875)
  line L8179 (-32.0085, 236.5375) -> (-26.5092, 246.0625)
  line L8180 (-12.7611, 266.7) -> (-23.7596, 266.7)
  line L8181 (-23.7596, 266.7) -> (-29.2589, 257.175)
  line L8182 (-29.2589, 257.175) -> (-23.7596, 247.65)
  line L8183 (-23.7596, 247.65) -> (-12.7611, 247.65)
  line L8184 (-7.2618, 257.175) -> (-12.7611, 266.7)
  line L8185 (-12.7611, 247.65) -> (-7.2618, 257.175)
  line L8186 (6.4863, 277.8125) -> (-4.5122, 277.8125)
  line L8187 (-4.5122, 277.8125) -> (-10.0114, 268.2875)
  line L8188 (-10.0114, 268.2875) -> (-4.5122, 258.7625)
  line L8189 (-4.5122, 258.7625) -> (6.4863, 258.7625)
  line L8190 (11.9856, 268.2875) -> (6.4863, 277.8125)
  line L8191 (6.4863, 258.7625) -> (11.9856, 268.2875)
  line L8192 (25.7337, 288.925) -> (14.7352, 288.925)
  line L8193 (14.7352, 288.925) -> (9.236, 279.4)
  line L8194 (9.236, 279.4) -> (14.7352, 269.875)
  line L8195 (14.7352, 269.875) -> (25.7337, 269.875)
  line L8196 (31.233, 279.4) -> (25.7337, 288.925)
  line L8197 (25.7337, 269.875) -> (31.233, 279.4)
  line L8198 (44.9812, 300.0375) -> (33.9826, 300.0375)
  line L8199 (33.9826, 300.0375) -> (28.4834, 290.5125)
  line L8200 (28.4834, 290.5125) -> (33.9826, 280.9875)
  line L8201 (33.9826, 280.9875) -> (44.9812, 280.9875)
  line L8202 (50.4804, 290.5125) -> (44.9812, 300.0375)
  line L8203 (44.9812, 280.9875) -> (50.4804, 290.5125)
  line L8204 (64.2286, 311.15) -> (53.2301, 311.15)
  line L8205 (53.2301, 311.15) -> (47.7308, 301.625)
  line L8206 (47.7308, 301.625) -> (53.2301, 292.1)
  line L8207 (53.2301, 292.1) -> (64.2286, 292.1)
  line L8208 (69.7278, 301.625) -> (64.2286, 311.15)
  line L8209 (64.2286, 292.1) -> (69.7278, 301.625)
  line L8210 (83.476, 322.2625) -> (72.4775, 322.2625)
  line L8211 (72.4775, 322.2625) -> (66.9782, 312.7375)
  line L8212 (66.9782, 312.7375) -> (72.4775, 303.2125)
  line L8213 (72.4775, 303.2125) -> (83.476, 303.2125)
  line L8214 (88.9753, 312.7375) -> (83.476, 322.2625)
  line L8215 (83.476, 303.2125) -> (88.9753, 312.7375)
  line L8216 (102.7234, 333.375) -> (91.7249, 333.375)
  line L8217 (91.7249, 333.375) -> (86.2256, 323.85)
  line L8218 (86.2256, 323.85) -> (91.7249, 314.325)
  line L8219 (91.7249, 314.325) -> (102.7234, 314.325)
  line L8220 (108.2227, 323.85) -> (102.7234, 333.375)
  line L8221 (102.7234, 314.325) -> (108.2227, 323.85)
  line L8222 (121.9708, 344.4875) -> (110.9723, 344.4875)
  line L8223 (110.9723, 344.4875) -> (105.473, 334.9625)
  line L8224 (105.473, 334.9625) -> (110.9723, 325.4375)
  line L8225 (110.9723, 325.4375) -> (121.9708, 325.4375)
  line L8226 (127.4701, 334.9625) -> (121.9708, 344.4875)
  line L8227 (121.9708, 325.4375) -> (127.4701, 334.9625)
  line L8228 (141.2182, 355.6) -> (130.2197, 355.6)
  line L8229 (130.2197, 355.6) -> (124.7205, 346.075)
  line L8230 (124.7205, 346.075) -> (130.2197, 336.55)
  line L8231 (130.2197, 336.55) -> (141.2182, 336.55)
  line L8232 (146.7175, 346.075) -> (141.2182, 355.6)
  line L8233 (141.2182, 336.55) -> (146.7175, 346.075)
  line L8234 (160.4657, 366.7125) -> (149.4671, 366.7125)
  line L8235 (149.4671, 366.7125) -> (143.9679, 357.1875)
  line L8236 (143.9679, 357.1875) -> (149.4671, 347.6625)
  line L8237 (149.4671, 347.6625) -> (160.4657, 347.6625)
  line L8238 (165.9649, 357.1875) -> (160.4657, 366.7125)
  line L8239 (160.4657, 347.6625) -> (165.9649, 357.1875)
  line L8240 (179.7131, 377.825) -> (168.7145, 377.825)
  line L8241 (168.7145, 377.825) -> (163.2153, 368.3)
  line L8242 (163.2153, 368.3) -> (168.7145, 358.775)
  line L8243 (168.7145, 358.775) -> (179.7131, 358.775)
  line L8244 (185.2123, 368.3) -> (179.7131, 377.825)
  line L8245 (179.7131, 358.775) -> (185.2123, 368.3)
  line L8246 (198.9605, 388.9375) -> (187.962, 388.9375)
  line L8247 (187.962, 388.9375) -> (182.4627, 379.4125)